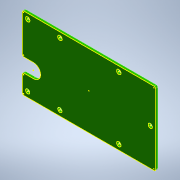
# Autodesk Inventor part: USB_PROG_PCB
Saved by Autodesk Inventor 2021 (Build 250183000, 183)
## iProperties
Created: 2020-02-27
Part Number: USB_PROG_PCB
Material: Generic
Document SubType Name: Modeling
Designer: lgnds
Density: 1 g/cm^3
Appearance: Default
Author: lgnds
Autodesk Inventor part; units mm, degrees
ref_plane "YZ Plane" through (0, 0, 0) normal (1, 0, 0) x (0, 1, 0)
ref_plane "XZ Plane" through (0, 0, 0) normal (0, 1, 0) x (-1, 0, 0)
ref_plane "XY Plane" through (0, 0, 0) normal (0, 0, 1) x (1, 0, 0)
sketch "Sketch1" plane through (0, 0, 0) normal (0, 0, 1) x (1, 0, 0)
  line L0 (-48.25, -26.8035) -> (48.25, -26.8035)
  line L1 (48.25, -26.8035) -> (48.25, 26.8035)
  line L2 (48.25, 26.8035) -> (-48.25, 26.8035)
  line L3 (-48.25, 26.8035) -> (-48.25, -26.8035)
  line L4 (-48.25, -26.8035) -> (48.25, 26.8035) construction
  line L5 (48.25, -26.8035) -> (-48.25, 26.8035) construction
  circle A0 centre (-43.75, 22.3035) radius 1.6
  circle A1 centre (-43.75, -22.3035) radius 1.6
  line L6 (-43.75, 22.3035) -> (54.6493, 22.3035) construction
  circle A2 centre (-20.75, 22.3035) radius 1.6
  circle A3 centre (21.25, 22.3035) radius 1.6
  line L7 (-68.8299, 0) -> (75.2292, 0) construction
  circle A4 centre (43.75, 0.1965) radius 1.6
  line L8 (-48.25, 26.8035) -> (48.25, -26.8035) construction
  line L9 (48.25, 26.8035) -> (-48.25, -26.8035) construction
  line L10 (-43.75, -22.3035) -> (54.6493, -22.3035) construction
  circle A5 centre (-20.75, -22.3035) radius 1.6
  circle A6 centre (21.25, -22.3035) radius 1.6
  point P0 (0, 0)
  dimension "d0" = 96.5
  dimension "d1" = 53.607
  dimension "d2" = 3.2
  dimension "d3" = 3.2
  dimension "d4" = 4.5
  dimension "d5" = 4.5
  dimension "d6" = 4.5
  dimension "d7" = 4.5
  dimension "d23" = 3.2
  dimension "d24" = 3.2
  dimension "d25" = 23
  dimension "d26" = 42
  dimension "d27" = 4.5
  dimension "d28" = 3.2
  dimension "d37" = 27
  constraints: 20 end point, 8 symmetric about line, 7 centre point, 4 point on line, 2 horizontal, 2 midpoint, 2 parallel, 1 perpendicular, 2 other
  measures "d0" distance of L1.end L2.end
  measures "d1" distance between parallel lines of L2 L0
  measures "d2" diameter of A0
  measures "d3" diameter of A1
  measures "d4" distance from line of L2 L6.start
  measures "d5" distance from line of L3 L6.start
  measures "d6" distance from line of L3 A1.centre
  measures "d7" distance from line of L0 A1.centre
  measures "d23" diameter of A2
  measures "d24" diameter of A3
  measures "d25" distance of L6.start A2.centre
  measures "d26" distance of A3.centre A2.centre
  measures "d27" distance from line of L1 A4.centre
  measures "d28" diameter of A4
  measures "d37" distance from line of L0 A4.centre
extrude "Extrusion1" add sketch "Sketch1" along normal blind 1.6
sketch "Sketch4" plane through (0, 0, 1.6) normal (0, 0, 1) x (1, 0, 0)
  arc A0 (-39.55, -12.3035) -> (-39.55, -2.3035) centre (-39.55, -7.3035) ccw
  line L0 (-48.25, -26.8035) -> (48.25, -26.8035) projected
  line L1 (-48.25, 26.8035) -> (-48.25, -26.8035) construction
  line L2 (-39.55, -2.3035) -> (-48.25, -2.3035)
  line L3 (-39.55, -12.3035) -> (-48.25, -12.3035)
  line L4 (-48.25, -2.3035) -> (-48.25, -12.3035)
  line L5 (-48.25, 26.8035) -> (-48.25, -26.8035) projected
  point P0 (0, 0)
  dimension "d29" = 19.5
  dimension "d30" = 8.7
  dimension "d31" = 10
  constraints: 6 end point, 2 point on circle, 2 point on line, 2 tangent, 1 centre point, 1 collinear, 1 parallel, 1 perpendicular
  measures "d29" distance from line of A0.centre L0
  measures "d30" distance from line of L1 A0.centre
  measures "d31" diameter of A0
extrude "Extrusion3" cut sketch "Sketch4" against normal up to next
thicken "Thicken1" operation add thickness 0.75 both sides no extend neighbours yes toward (0, 1, 0) faces at (-16.0833, -26.8035, 0.5333) (48.25, -8.9345, 0.5333) (16.0833, 26.8035, 0.5333) (-48.25, 17.1012, 0.5333) (-48.25, -21.9702, 1.0667)
fillet "Fillet1" radius 1 6 edges at (-47.5, 26.0535, 0.8) (47.5, 26.0535, 0.8) (47.5, -26.0535, 0.8) (-47.5, -26.0535, 0.8) (-47.5, -12.3035, 0.8) (-47.5, -2.3035, 0.8)
sketch "OUTLINE" plane through (0, 0, 1.6) normal (0, 0, 1) x (1, 0, 0)
  line L0 (46.5, 26.0535) -> (-46.5, 26.0535) projected
  arc A0 (47.5, 25.0535) -> (46.5, 26.0535) centre (46.5, 25.0535) ccw projected
  line L1 (47.5, -25.0535) -> (47.5, 25.0535) projected
  arc A1 (46.5, -26.0535) -> (47.5, -25.0535) centre (46.5, -25.0535) ccw projected
  line L2 (-46.5, -26.0535) -> (46.5, -26.0535) projected
  arc A2 (-47.5, -25.0535) -> (-46.5, -26.0535) centre (-46.5, -25.0535) ccw projected
  line L3 (-47.5, -13.3035) -> (-47.5, -25.0535) projected
  arc A3 (-46.5, -12.3035) -> (-47.5, -13.3035) centre (-46.5, -13.3035) ccw projected
  line L4 (-39.55, -12.3035) -> (-46.5, -12.3035) projected
  arc A4 (-39.55, -12.3035) -> (-39.55, -2.3035) centre (-39.55, -7.3035) ccw projected
  line L5 (-46.5, -2.3035) -> (-39.55, -2.3035) projected
  arc A5 (-47.5, -1.3035) -> (-46.5, -2.3035) centre (-46.5, -1.3035) ccw projected
  line L6 (-47.5, 25.0535) -> (-47.5, -1.3035) projected
  arc A6 (-46.5, 26.0535) -> (-47.5, 25.0535) centre (-46.5, 25.0535) ccw projected
  point P0 (0, 0)
sketch "EXTRA" plane through (0, 0, 1.6) normal (0, 0, 1) x (1, 0, 0)
  circle A0 centre (-43.75, 22.3035) radius 1.6 projected
  circle A1 centre (-20.75, 22.3035) radius 1.6 projected
  circle A2 centre (21.25, 22.3035) radius 1.6 projected
  circle A3 centre (43.75, 0.1965) radius 1.5 projected
  circle A4 centre (21.25, -22.3035) radius 1.6 projected
  circle A5 centre (-20.75, -22.3035) radius 1.5 projected
  circle A6 centre (-43.75, -22.3035) radius 1.5 projected
  point P0 (0, 0)
equation "\"d3\" = d2"
equation "\"d6\" = d4"
equation "\"d7\" = d6"
equation "\"d23\" = d2"
equation "\"d24\" = d2"
equation "\"d27\" = d5"
equation "\"d28\" = d2"
body "Solid1"
